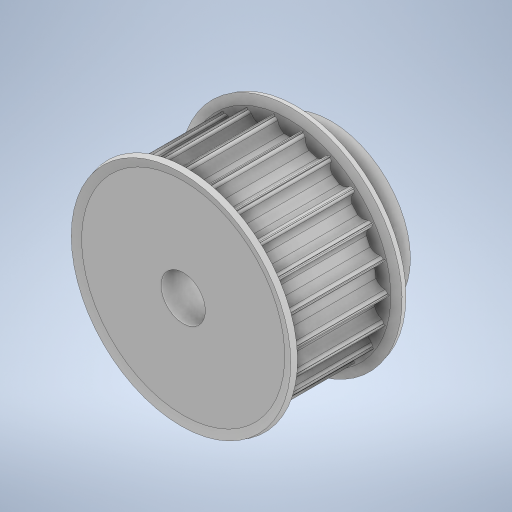
# Autodesk Inventor part: Engine Belt Wheel
Saved by Autodesk Inventor 2024 (Build 280153000, 153)
## iProperties
Created: 2023-07-01
Part Number: Engine Belt Wheel
Material: Generic
Document SubType Name: Modeling
Designer: vilas
Density: 1 g/cm^3
Appearance: Default
Author: vilas
Autodesk Inventor part; units mm, degrees
ref_plane "YZ Plane" through (0, 0, 0) normal (1, 0, 0) x (0, 1, 0)
ref_plane "XZ Plane" through (0, 0, 0) normal (0, 1, 0) x (-1, 0, 0)
ref_plane "XY Plane" through (0, 0, 0) normal (0, 0, 1) x (1, 0, 0)
sketch "Sketch1" plane through (0, 0, 0) normal (1, 0, 0) x (0, 1, 0)
  line L0 (6, 0) -> (27.25, 0)
  line L1 (27.25, 0) -> (27.25, -30)
  line L2 (27.25, -30) -> (21.5, -30)
  line L3 (21.5, -30) -> (21.5, -40)
  line L4 (21.5, -40) -> (6, -40)
  line L5 (6, -40) -> (6, 0)
  line L6 (0, -48) -> (0, 8) projected
  point P0 (0, 0)
  dimension "d0" = 6
  dimension "d1" = 21.25
  dimension "d2" = 30
  dimension "d4" = 15.5
  dimension "d5" = 10
  constraints: 12 end point, 5 perpendicular, 1 horizontal
  measures "d0" distance from line of point (0, 0) L5
  measures "d1" distance of L0.start L0.end
  measures "d2" distance of L0.end L1.end
  measures "d4" distance of L3.end L4.end
  measures "d5" distance of L2.end L3.end
revolve "Revolution1" add sketch "Sketch1" angle 360 about axis through (0, 0, -10) along (0, 0, 1)
sketch "Sketch2" plane through (0, 0, 0) normal (0, 0, 1) x (1, 0, 0)
  line L0 (0, 0) -> (0, 27.5) construction
  line L1 (-3.75, 28.5) -> (3.75, 28.5)
  line L2 (3.75, 28.5) -> (3.75, 26.5)
  line L3 (-3.75, 26.5) -> (-3.75, 28.5)
  line L4 (-3.75, 28.5) -> (3.75, 26.5) construction
  line L5 (3.75, 28.5) -> (-3.75, 26.5) construction
  arc A0 (-2.9394, 25.9) -> (2.9394, 25.9) centre (0, 26.5) ccw
  line L6 (3.75, 26.5) -> (3.6742, 26.5)
  line L7 (-3.6742, 26.5) -> (-3.75, 26.5)
  arc A1 (-2.9394, 25.9) -> (-3.6742, 26.5) centre (-3.6742, 25.75) ccw
  arc A2 (3.6742, 26.5) -> (2.9394, 25.9) centre (3.6742, 25.75) ccw
  line L8 (-1.199, 23.75) -> (1.199, 23.75)
  point P0 (-3, 26.5)
  point P1 (3, 26.5)
  dimension "d7" = 27.5
  dimension "d8" = 7.5
  dimension "d9" = 2
  dimension "d10" = 3
  dimension "d11" = 0.75
  dimension "d12" = 0.75
  dimension "d13" = 0.75
  dimension "d14" = 2.75
  constraints: 18 end point, 10 point on circle, 4 tangent, 3 centre point, 3 parallel, 2 horizontal, 2 midpoint, 2 point on line, 1 equal radius, 1 perpendicular, 1 vertical
  measures "d7" distance of L0.start L0.end
  measures "d8" distance of L2.end L3.start
  measures "d9" distance of L1.end L2.end
  measures "d10" radius of A0
  measures "d11" distance of point (-3, 26.5) L3.start
  measures "d12" distance of L2.end point (3, 26.5)
  measures "d13" radius of A1
  measures "d14" distance from line of A0.centre L8
extrude "Extrusion1" cut sketch "Sketch2" against normal through all contours L1 L2 L6 A2 A0 L8 A1 L7 L3
pattern_circular "Circular Pattern1" count 22 over 360 about axis through (0, 0, -10) along (0, 0, 1) of "Extrusion1"
sketch "Sketch3" plane through (0, 0, 0) normal (1, 0, 0) x (0, 1, 0)
  line L0 (22.6907, 0) -> (27.6907, 0)
  line L1 (27.6907, 0) -> (27.6907, -1.5)
  line L2 (27.6907, -1.5) -> (22.6907, -1.5)
  line L3 (22.6907, -1.5) -> (22.6907, 0)
  line L4 (27.6907, -1.5) -> (30.0907, -0.8569)
  line L5 (30.0907, -0.8569) -> (29.7025, 0.592)
  line L6 (29.7025, 0.592) -> (27.3025, -0.0511)
  line L7 (27.3025, -0.0511) -> (27.6907, -1.5)
  line L8 (27.6907, -1.5) -> (30.1754, -1.5) construction
  line L9 (26.9907, 0) -> (26.9907, -30) projected
  line L10 (23.75, 0) -> (25.9, 0) projected
  line L11 (26.9907, -15) -> (-26.9907, -15) construction
  line L12 (-26.9907, -30) -> (-26.9907, 0) construction
  line L13 (22.6907, -30) -> (27.6907, -30)
  line L14 (27.6907, -30) -> (27.6907, -28.5)
  line L15 (27.6907, -28.5) -> (22.6907, -28.5)
  line L16 (22.6907, -28.5) -> (22.6907, -30)
  line L17 (27.6907, -28.5) -> (30.0907, -29.1431)
  line L18 (30.0907, -29.1431) -> (29.7025, -30.592)
  line L19 (29.7025, -30.592) -> (27.3025, -29.9489)
  line L20 (27.3025, -29.9489) -> (27.6907, -28.5)
  line L21 (27.6907, -28.5) -> (30.1754, -28.5) construction
  line L22 (23.75, -30) -> (25.9, -30)
  line L23 (0, -48.1184) -> (0, 8.7104) projected
  point P0 (0, 0)
  point P1 (27.4933, 0)
  point P2 (27.4933, -30)
  dimension "d20" = 5
  dimension "d21" = 1.5
  dimension "d22" = 15
  dimension "d23" = 1.5
  dimension "d24" = 2.4
  dimension "d25" = 0.7
  dimension "d26" = 0
  constraints: 40 end point, 10 symmetric about line, 4 parallel, 2 horizontal, 2 midpoint, 2 perpendicular, 1 equal length
  measures "d20" distance of L1.end L2.end
  measures "d21" distance of L0.end L1.end
  measures "d22" angle of L8 L4
  measures "d23" distance of L5.end L4.end
  measures "d24" horizontal distance of L1.end L4.end
  measures "d25" distance between parallel lines of L9 L1
  measures "d26" distance between parallel lines of L0 L10
revolve "Revolution2" add sketch "Sketch3" angle 360 about axis through (0, 0, -10) along (0, 0, 1)
body "Solid1"
